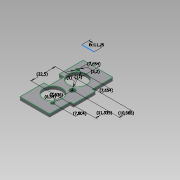
# Autodesk Inventor part: srf
Saved by Autodesk Inventor 2015 SP1 (Build 190203100, 203)
## iProperties
Created: 2014-12-05
Part Number: srf
Material: Generic
Document SubType Name: Modeling
Designer: Yosua
Density: 1 g/cm^3
Appearance: Default
Author: Yosua
Autodesk Inventor part; units mm, degrees
ref_plane "YZ Plane" through (0, 0, 0) normal (1, 0, 0) x (0, 1, 0)
ref_plane "XZ Plane" through (0, 0, 0) normal (0, 1, 0) x (-1, 0, 0)
ref_plane "XY Plane" through (0, 0, 0) normal (0, 0, 1) x (1, 0, 0)
sketch "Sketch1" plane through (0, 0, 0) normal (0, 0, 1) x (1, 0, 0)
  circle A0 centre (-14.6869, 39.4735) radius 8.5
  circle A1 centre (-22.3409, 47.1275) radius 1.6
  circle A2 centre (-7.0512, 9.17) radius 1.6
  circle A3 centre (-8.1473, 28.508) radius 2.5
  circle A4 centre (-14.6869, 16.9735) radius 8.5
  line L0 (0, 28.315) -> (0, -0.685)
  line L1 (0, -0.685) -> (-27.2, -0.685)
  line L2 (-27.2, -0.685) -> (0, -0.685)
  line L3 (0, -0.685) -> (0, 57.315)
  line L4 (0, 57.315) -> (-27.2, 57.315)
  line L5 (-27.2, 57.315) -> (-27.2, -0.685)
  line L6 (0, 28.315) -> (0, 38.315)
  line L7 (0, 38.315) -> (3, 38.315)
  line L8 (3, 38.315) -> (3, 18.315)
  line L9 (3, 18.315) -> (0, 18.315)
  line L10 (-14.6869, 39.4735) -> (-14.6869, 28.315)
  line L11 (-14.6869, 28.315) -> (-22.6869, 28.315)
  line L12 (-22.6869, 28.315) -> (-22.6869, 21.315)
  line L13 (-22.6869, 21.315) -> (-22.6869, 35.315)
  line L14 (-22.6869, 35.315) -> (-27.2, 35.315)
  line L15 (-22.6869, 21.315) -> (-27.2, 21.315)
  point P0 (0, 0)
  point P1 (-5.6598, 20.3223)
  dimension "d1" = 29
  dimension "d2" = 58
  dimension "d3" = 10
  dimension "d4" = 3
  dimension "d5" = 20
  dimension "d10" = 8
  dimension "d11" = 7
  dimension "d12" = 14
  constraints: 32 end point, 8 perpendicular, 5 centre point, 4 parallel, 4 point on line, 1 collinear, 1 horizontal
  measures "d1" distance of L0.start L0.end
  measures "d2" distance of L3.end L2.end
  measures "d3" distance of L0.start L6.end
  measures "d4" distance of L6.end L7.end
  measures "d5" distance of L7.end L8.end
  measures "d10" distance of L10.end L11.end
  measures "d11" distance of L11.end L12.end
  measures "d12" distance of L12.end L13.end
extrude "Extrusion2" add sketch "Sketch1" along normal blind 3 contours L13 L14 L5 L4 L3 L0 L1 L15 L12 | L0 L3 L7 L8 L9
sketch "Sketch2" plane through (0, 0, 3) normal (0, 0, 1) x (1, 0, 0)
  circle A0 centre (-14.6869, 16.9735) radius 8.5 projected
  circle A1 centre (-14.6869, 39.4735) radius 8.5 projected
  circle A2 centre (-8.1473, 28.508) radius 2.5 projected
  circle A3 centre (-7.0512, 9.17) radius 1.6 projected
  circle A4 centre (-22.3409, 47.1275) radius 1.6 projected
  line L0 (0, 18.315) -> (3, 18.315) projected
  line L1 (3, 18.315) -> (3, 38.315) projected
  line L2 (3, 38.315) -> (0, 38.315) projected
  line L3 (0, 38.315) -> (0, 57.315) projected
  line L4 (0, 57.315) -> (-27.2, 57.315) projected
  line L5 (-27.2, 57.315) -> (-27.2, 35.315) projected
  line L6 (-27.2, 35.315) -> (-22.6869, 35.315) projected
  line L7 (-22.6869, 35.315) -> (-22.6869, 21.315) projected
  line L8 (-22.6869, 21.315) -> (-27.2, 21.315) projected
  line L9 (-27.2, 21.315) -> (-27.2, -0.685) projected
  line L10 (-27.2, -0.685) -> (0, -0.685) projected
  line L11 (0, -0.685) -> (0, 18.315) projected
  line L12 (-40, 69) -> (-28.75, 69)
  point P0 (0, 0)
  dimension "d15" = 17
  dimension "d16" = 3.2
  dimension "d17" = 5
  dimension "d18" = 22.5
  dimension "d19" = 7.654
  dimension "d20" = 7.654
  dimension "d21" = 7.6357
  dimension "d22" = 7.8035
  dimension "d23" = 6.5396
  dimension "d24" = 11.5345
  dimension "d25" = 10.9655
  dimension "d26" = 11.25
  constraints: 2 end point, 1 horizontal
  measures "d15" diameter of A1
  measures "d16" diameter of A4
  measures "d17" diameter of A2
  measures "d18" distance of A0.centre A1.centre
  measures "d19" horizontal distance of A4.centre A1.centre
  measures "d20" horizontal distance of A1.centre A4.centre
  measures "d21" horizontal distance of A3.centre A0.centre
  measures "d22" vertical distance of A3.centre A0.centre
  measures "d23" horizontal distance of A0.centre A2.centre
  measures "d24" vertical distance of A2.centre A0.centre
  measures "d25" vertical distance of A2.centre A1.centre
  measures "d26" distance of L12.start L12.end
equation "\"d26\" = 0.5 * d24 + 0.5 * d25"
body "Solid2"
